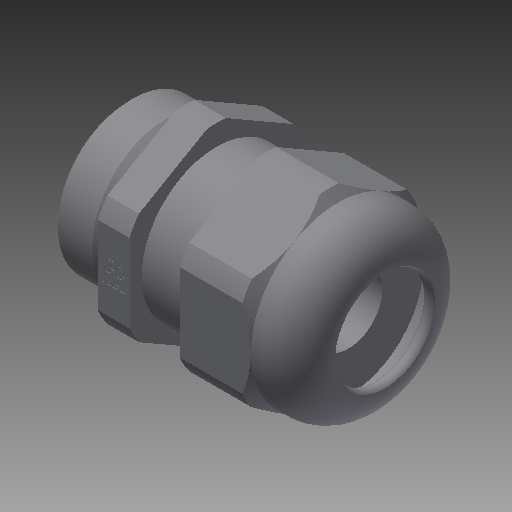
# Autodesk Inventor part: SKINTOP ST PG 21      Art. Nr. 53015050(F=13) Kunststoff
Saved by Autodesk Inventor 2019.3 (Build 233278000, 278)
## iProperties
Category: PARTsolutions
Company: LAPP
Created: 2018-12-14
Part Number: SKINTOP ST PG 21      Art. Nr. 53015050(F=13) Kunststoff
Material: Generic
Catalog Web Link: www.cadenas.de
Description: SKINTOP® ST-Cable gland plastic
Vendor: LAPP
Document SubType Name: Modeling
Designer: psadmin
Manufacturer: LAPP
Mass: 28.7646 g
Surface Area: 95.472 cm^2
Volume: 28.7646 cm^3
Density: 1 g/cm^3
Appearance: PSOLRGB-175-175-175
PSOL_IDENT_0: {$CADENAS_DATA\23d-libs\lapp_kabel\skintop_kabelverschraubungen\skintop_kabelverschraubungen_polyami
PSOL_IDENT_1: d_pg\skintop_kabelverschraubungen_polyamid_pg\st_pg.prj},232 {VTYP=3D},{NB=SKINTOP ST PG 21      Art
PSOL_IDENT_2: . Nr. 53015050(F=13)},{LINA=SKINTOP ST PG 21      Art. Nr. 53015050},{NN=SKINTOP® ST},{DATE=06.12.20
PSOL_IDENT_3: 18 13:21:11},{GEOMDATE=18.12.2013 09:14:44},{VERSION=},{LINEID=160},{WBVAR=F},{WBNUMERIC=F}  {NB=SKI
PSOL_IDENT_4: NTOP ST PG 21      Art. Nr. 53015050(F=13)},{LINA=SKINTOP ST PG 21      Art. Nr. 53015050},{KT=DUMMY
PSOL_IDENT_5: },{IDNR=},{ATN=53015050},{PG=PG 21},{ID=0.000},{RS=0.000},{FMIN=13.0},{FMAX=18.0},{F=13},{NDM=28.3},
PSOL_IDENT_6: {X=9.5},{SW=33},{A=36.2},{C=49.0},{D=11.0},{E=22.5},{H=13.5},{J=7.0},{K=6.0},{L=28.4},{XMAX=9.5},{RA
PSOL_IDENT_7: L7001=X},{RAL7035=},{RAL9005=},{MATERIAL=Kunststoff},{VPE=MIN}
NN: SKINTOP® ST
NT: Cable gland plastic
NB: SKINTOP® ST PG 21      Art. Nr. 53015050(F=13)
NBSYN: SKINTOP® ST $PG.      Art. Nr. $ATN.(F=$F.)
LINA: SKINTOP® ST PG 21      Art. Nr. 53015050
ATN: 53015050
PG: PG 21
FMIN: 13
FMAX: 18
F: 13
SW: 33
A: 36.2
C: 49
D: 11
RAL7001: X
MATERIAL: Plastic
VPE: 0
SUPPLIER: LAPP
ARTICLENO: SKINTOP ST PG 21      Art. Nr. 53015050(F=13)
BOMINFO: SKINTOP ST PG 21      Art. Nr. 53015050
CREATOR: CADENAS GmbH
Title: SKINTOP ST PG 21      Art. Nr. 53015050
Author: Cadenas PARTsolutions
Comments: Cable gland plastic
Autodesk Inventor part; units mm, degrees
ref_plane "YZ Plane" through (0, 0, 0) normal (1, 0, 0) x (0, 1, 0)
ref_plane "XZ Plane" through (0, 0, 0) normal (0, 1, 0) x (-1, 0, 0)
ref_plane "XY Plane" through (0, 0, 0) normal (0, 0, 1) x (1, 0, 0)
sketch "Sketch_1" plane through (0, 0, 0) normal (0, 0, 1) x (1, 0, 0)
  line L0 (49, 0) -> (0, 0)
  line L1 (0, 12.6775) -> (0, 7.265)
  arc A0 (0, 7.265) -> (0.765, 6.5) centre (0.765, 7.265) ccw
  line L2 (0.765, 6.5) -> (42, 6.5)
  line L3 (42, 6.5) -> (42, 14.2)
  arc A1 (46.6897, 9.8103) -> (42, 14.2) centre (42, 9.5) ccw
  arc A2 (46.6897, 9.8103) -> (49, 9.5) centre (47.9481, 10.4239) ccw
  arc A3 (49, 9.5) -> (42, 16.5) centre (42, 9.5) ccw
  line L4 (42, 16.5) -> (40, 16.5)
  line L5 (40, 16.5) -> (34.5, 22)
  line L6 (34.5, 22) -> (26.5, 22)
  line L7 (26.5, 22) -> (26.5, 14.2)
  line L8 (26.5, 14.2) -> (17, 14.2)
  line L9 (17, 14.2) -> (17, 22)
  line L10 (17, 22) -> (11, 22)
  line L11 (11, 22) -> (11, 13.4425)
  line L12 (11, 13.4425) -> (8.8, 13.4425)
  line L13 (8.8, 13.4425) -> (7.5746, 14.15)
  line L14 (7.5746, 14.15) -> (1.1, 14.15)
  line L15 (1.1, 14.15) -> (1.1, 13.4425)
  line L16 (1.1, 13.4425) -> (0.765, 13.4425)
  arc A4 (0.765, 13.4425) -> (0, 12.6775) centre (0.765, 12.6775) ccw
  constraints: 34 end point, 10 point on circle, 5 centre point
revolve "Revolution1" add sketch "Sketch_1" angle 360 about axis through (49, 0, 0) along (-1, 0, 0)
sketch "Sketch_2" plane through (11, 0, 0) normal (1, 0, 0) x (0, 0, -1)
  line L0 (-33, 33) -> (-33, -33)
  line L1 (-33, -33) -> (33, -33)
  line L2 (33, -33) -> (33, 33)
  line L3 (33, 33) -> (-33, 33)
  arc A0 (-16.5, -7.4404) -> (-14.6936, -10.5692) centre (0, 0) ccw
  line L4 (-14.6936, -10.5692) -> (-1.8064, -18.0096)
  arc A1 (-1.8064, -18.0096) -> (1.8064, -18.0096) centre (0, 0) ccw
  line L5 (1.8064, -18.0096) -> (14.6936, -10.5692)
  arc A2 (14.6936, -10.5692) -> (16.5, -7.4404) centre (0, 0) ccw
  line L6 (16.5, -7.4404) -> (16.5, 7.4404)
  arc A3 (16.5, 7.4404) -> (14.6936, 10.5692) centre (0, 0) ccw
  line L7 (14.6936, 10.5692) -> (1.8064, 18.0096)
  arc A4 (1.8064, 18.0096) -> (-1.8064, 18.0096) centre (0, 0) ccw
  line L8 (-1.8064, 18.0096) -> (-14.6936, 10.5692)
  arc A5 (-14.6936, 10.5692) -> (-16.5, 7.4404) centre (0, 0) ccw
  line L9 (-16.5, 7.4404) -> (-16.5, -7.4404)
  constraints: 20 end point, 12 point on circle, 6 centre point
extrude "Extrusion1" cut sketch "Sketch_2" along normal blind 49
sketch "Skizze_1" plane through (0, 0, 16.5) normal (0, 0, 1) x (1, 0, 0)
  line L0 (11.8, 2.2) -> (11.8, -2.2)
  line L1 (11.8, -2.2) -> (16.2, -2.2)
  line L2 (16.2, -2.2) -> (16.2, 2.2)
  line L3 (16.2, 2.2) -> (11.8, 2.2)
  arc A0 (12.0456, 0.4247) -> (12.6685, -1.4924) centre (14, 0) ccw
  line L4 (12.6685, -1.4924) -> (12.759, -1.3678)
  arc A1 (13.0827, -1.6029) -> (12.759, -1.3678) centre (13.2947, -0.9708) ccw
  line L5 (13.0827, -1.6029) -> (12.9921, -1.7275)
  arc A2 (12.9921, -1.7275) -> (15.0079, -1.7275) centre (14, 0) ccw
  line L6 (15.0079, -1.7275) -> (14.9173, -1.6029)
  arc A3 (15.241, -1.3678) -> (14.9173, -1.6029) centre (14.7053, -0.9708) ccw
  line L7 (15.241, -1.3678) -> (15.3315, -1.4924)
  arc A4 (15.3315, -1.4924) -> (15.9544, 0.4247) centre (14, 0) ccw
  line L8 (15.9544, 0.4247) -> (15.8079, 0.3771)
  arc A5 (15.6843, 0.7576) -> (15.8079, 0.3771) centre (15.1413, 0.3708) ccw
  line L9 (15.6843, 0.7576) -> (15.8308, 0.8051)
  arc A6 (15.8308, 0.8051) -> (14.2, 1.99) centre (14, 0) ccw
  line L10 (14.2, 1.99) -> (14.2, 1.836)
  arc A7 (13.8, 1.836) -> (14.2, 1.836) centre (14, 1.2) ccw
  line L11 (13.8, 1.836) -> (13.8, 1.99)
  arc A8 (13.8, 1.99) -> (12.1692, 0.8051) centre (14, 0) ccw
  line L12 (12.1692, 0.8051) -> (12.3157, 0.7576)
  arc A9 (12.1921, 0.3771) -> (12.3157, 0.7576) centre (12.8587, 0.3708) ccw
  line L13 (12.1921, 0.3771) -> (12.0456, 0.4247)
  constraints: 28 end point, 20 point on circle, 10 centre point
extrude "Extrusion2" cut sketch "Skizze_1" against normal blind 0.066
body "Solid1"
